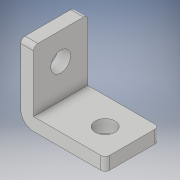
# Autodesk Inventor part: elbow
Saved by Autodesk Inventor 2017 (Build 210142000, 142)
## iProperties
Created: 2016-12-07
Part Number: elbow
Material: Generic
Document SubType Name: Modeling
Designer: PLTW
Density: 1 g/cm^3
Appearance: Default
Author: PLTW
Autodesk Inventor part; units mm, degrees
ref_plane "YZ Plane" through (0, 0, 0) normal (1, 0, 0) x (0, 1, 0)
ref_plane "XZ Plane" through (0, 0, 0) normal (0, 1, 0) x (-1, 0, 0)
ref_plane "XY Plane" through (0, 0, 0) normal (0, 0, 1) x (1, 0, 0)
sketch "Sketch2" plane through (0, 0, 0) normal (0, 0, 1) x (1, 0, 0)
  line L0 (0, 8.763) -> (1.524, 8.763)
  line L1 (1.524, 8.763) -> (1.524, 1.524)
  line L2 (1.524, 1.524) -> (0, 1.524)
  line L3 (0, 1.524) -> (0, 8.763)
  line L4 (1.524, 1.524) -> (9.9822, 1.524)
  line L5 (9.9822, 1.524) -> (9.9822, 0)
  line L6 (9.9822, 0) -> (1.524, 0)
  line L7 (1.524, 0) -> (1.524, 1.524)
  arc A0 (0, 1.524) -> (1.524, 0) centre (1.524, 1.524) ccw
  point P0 (0, 0)
  dimension "d9" = 1.524
  dimension "d10" = 7.239
  dimension "d11" = 8.4582
  constraints: 16 end point, 4 parallel, 3 perpendicular, 2 horizontal, 2 point on circle, 1 centre point, 1 horizontal alignment, 1 tangent, 1 vertical alignment
  measures "d9" distance of L0.start L0.end
  measures "d10" distance between parallel lines of L4 L0
  measures "d11" distance of L1.end L4.end
extrude "Extrusion2" add sketch "Sketch2" along normal blind 6.4008
fillet "Fillet2" radius 0.508 4 edges at (0.762, 8.763, 6.4008) (0.762, 8.763, 0) (9.9822, 0.762, 6.4008) (9.9822, 0.762, 0)
sketch "Sketch3" plane through (1.524, 1.524, 6.4008) normal (0, 1, 0) x (1, 0, 0)
  circle A0 centre (5.2578, 3.2004) radius 1.1684
  line L0 (8.4582, 5.8928) -> (8.4582, 0.508) projected
  line L1 (7.9502, 0) -> (0, 0) projected
  point P0 (-1.524, 6.4008)
  point P1 (8.4582, 3.2004)
  dimension "d15" = 3.2004
  dimension "d16" = 3.2004
  dimension "d17" = 2.3368
  constraints: 1 centre point, 1 horizontal alignment, 1 midpoint
  measures "d15" distance from line of L0 A0.centre
  measures "d16" distance from line of L1 A0.centre
  measures "d17" diameter of A0
extrude "Extrusion3" cut sketch "Sketch3" against normal through all
sketch "Sketch4" plane through (1.524, 1.524, 6.4008) normal (1, 0, 0) x (0, 0, -1)
  circle A0 centre (3.2004, 4.0386) radius 1.1684
  line L0 (5.8928, 7.239) -> (0.508, 7.239) projected
  line L1 (6.4008, 0) -> (6.4008, 6.731) projected
  point P0 (6.4008, -1.524)
  point P1 (3.2004, 7.239)
  dimension "d20" = 3.2004
  dimension "d21" = 3.2004
  dimension "d22" = 2.3368
  constraints: 1 centre point, 1 midpoint, 1 vertical alignment
  measures "d20" distance from line of L1 A0.centre
  measures "d21" distance from line of L0 A0.centre
  measures "d22" diameter of A0
extrude "Extrusion4" cut sketch "Sketch4" against normal through all
equation "\"d15\" = d16"
equation "\"d21\" = d20"
body "Solid2"
